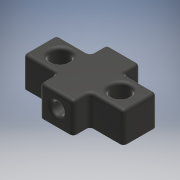
# Autodesk Inventor part: bed_spring_holder_v3
Saved by Autodesk Inventor 2018 (Build 220112000, 112)
## iProperties
Created: 2018-05-25
Part Number: bed_spring_holder_v3
Material: Plastic, Opaque Black
Document SubType Name: Modeling
Designer: Z. Deniz
Density: 0.952 g/cm^3
Appearance: Smooth - Black
Author: Z. Deniz
Autodesk Inventor part; units mm, degrees
ref_plane "YZ Plane" through (0, 0, 0) normal (1, 0, 0) x (0, 1, 0)
ref_plane "XZ Plane" through (0, 0, 0) normal (0, 1, 0) x (-1, 0, 0)
ref_plane "XY Plane" through (0, 0, 0) normal (0, 0, 1) x (1, 0, 0)
sketch "Sketch1" plane through (0, 0, 0) normal (1, 0, 0) x (0, 1, 0)
  line L0 (25, 0) -> (25, 9)
  line L1 (25, 9) -> (0, 9)
  line L2 (0, 9) -> (0, 0)
  line L3 (0, 0) -> (20, 0) construction
  line L4 (5, 0) -> (25, 0)
  line L5 (20, 9) -> (10, 9)
  line L6 (10, 9) -> (10, 0)
  line L7 (10, 0) -> (20, 0)
  line L8 (20, 0) -> (20, 9)
  line L9 (20, 9) -> (10, 0) construction
  line L10 (10, 9) -> (20, 0) construction
  line L11 (5, 0) -> (5, 9)
  line L12 (5, 0) -> (0, 0)
  point P0 (15, 4.5)
  dimension "d8" = 9
  dimension "d13" = 10
  dimension "d14" = 9
  dimension "d15" = 25
  dimension "d39" = 10
  dimension "d47" = 5
  constraints: 26 end point, 4 parallel, 3 horizontal, 3 perpendicular, 3 point on line, 2 midpoint, 1 collinear
  measures "d8" distance of L0.end L0.start
  measures "d13" distance of L7.end L6.end
  measures "d14" distance of L7.end L5.start
  measures "d15" distance between parallel lines of L2 L0
  measures "d39" distance between parallel lines of L6 L2
  measures "d47" distance between parallel lines of L2 L11
extrude "Extrusion1" add sketch "Sketch1" along normal mid plane 10 contours L4 L8 L1 L0 | L4 L11 L1 L6
extrude "Extrusion2" add sketch "Sketch1" along normal mid plane 30 contours L4 L6 L1 L8
sketch "Sketch8" plane through (-5, 5, 9) normal (0, 0, 1) x (1, 0, 0)
  circle A0 centre (-4, 10) radius 2.75
  line L0 (-10, 5) -> (-10, 15) projected
  line L1 (-10, 15) -> (0, 15) projected
  circle A1 centre (14, 10) radius 2.75
  line L2 (20, 15) -> (20, 5) projected
  line L3 (10, 15) -> (20, 15) projected
  point P0 (5, -5)
  dimension "d48" = 5.5
  dimension "d49" = 6
  dimension "d50" = 5
  dimension "d51" = 5.5
  dimension "d52" = 6
  dimension "d53" = 5
  constraints: 2 centre point
  measures "d48" diameter of A0
  measures "d49" distance from line of L0 A0.centre
  measures "d50" distance from line of L1 A0.centre
  measures "d51" diameter of A1
  measures "d52" distance from line of L2 A1.centre
  measures "d53" distance from line of L3 A1.centre
extrude "Extrusion8" cut sketch "Sketch8" against normal through all
sketch "Sketch9" plane through (-5, 25, 9) normal (0, 1, 0) x (1, 0, 0)
  circle A0 centre (5, 4.5) radius 1.75
  line L0 (0, 9) -> (10, 9) projected
  line L1 (10, 9) -> (10, 0) projected
  line L2 (0, 0) -> (0, 9) projected
  point P0 (5, 9)
  dimension "d56" = 3.5
  dimension "d57" = 4.5
  dimension "d58" = 10
  dimension "d59" = 5
  constraints: 1 centre point
  measures "d56" diameter of A0
  measures "d57" distance from line of L0 A0.centre
  measures "d58" distance between parallel lines of L1 L2
  measures "d59" distance from line of L2 A0.centre
extrude "Extrusion9" cut sketch "Sketch9" against normal through all
fillet "Fillet4" radius 1 28 edges at (0, 25, 9) (-10, 20, 9) (-5, 22.5, 9) (5, 22.5, 9) (10, 20, 9) (5, 25, 4.5) (5, 20, 4.5) (-5, 25, 4.5) (-5, 20, 4.5) (10, 10, 9) (15, 15, 9) (15, 20, 4.5) (15, 10, 4.5) (5, 5, 4.5) (5, 7.5, 9) (5, 10, 4.5) (0, 5, 9) (-5, 7.5, 9) (-5, 10, 4.5) (-10, 10, 9) (-15, 15, 9) (-5, 5, 4.5) (-15, 10, 4.5) (-15, 20, 4.5) (6.25, 15, 9) (-11.75, 15, 9) (-1.75, 5, 4.5) (-1.75, 25, 4.5)
equation "\"d52\" = d49"
equation "\"d59\" = 0.5 * d58"
body "Solid1"
